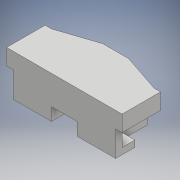
# Autodesk Inventor part: NewLaptopSupport
Saved by Autodesk Inventor 2017 (Build 210142000, 142)
## iProperties
Created: 2016-11-02
Part Number: NewLaptopSupport
Material: Generic
Document SubType Name: Modeling
Designer: Schmidty15
Density: 1 g/cm^3
Appearance: Default
Author: Schmidty15
Autodesk Inventor part; units mm, degrees
ref_plane "YZ Plane" through (0, 0, 0) normal (1, 0, 0) x (0, 1, 0)
ref_plane "XZ Plane" through (0, 0, 0) normal (0, 1, 0) x (-1, 0, 0)
ref_plane "XY Plane" through (0, 0, 0) normal (0, 0, 1) x (1, 0, 0)
sketch "Sketch1" plane through (0, 0, 0) normal (0, 1, 0) x (-1, 0, 0)
  line L0 (0, 0) -> (-160, 0)
  line L1 (-160, 0) -> (-160, 60)
  line L2 (-160, 60) -> (0, 60)
  line L3 (0, 60) -> (0, 0)
  dimension "d0" = 160
  dimension "d1" = 60
  constraints: 8 end point, 2 parallel, 1 horizontal, 1 perpendicular
  measures "d0" distance of L1.end L2.end
  measures "d1" distance of L0.end L1.end
extrude "Extrusion1" add sketch "Sketch1" along normal blind 80
sketch "Sketch2" plane through (0, 80, 0) normal (0, 1, 0) x (1, 0, 0)
  line L0 (160, 0) -> (0, 0) projected
  line L1 (160, 0) -> (150, 0)
  line L2 (150, 0) -> (150, -10)
  line L3 (150, -10) -> (160, -10)
  line L4 (160, -10) -> (160, 0)
  line L5 (160, -10) -> (0, -10)
  line L6 (0, -10) -> (0, -40)
  line L7 (0, -40) -> (160, -40)
  line L8 (160, -40) -> (160, -10)
  dimension "d4" = 10
  dimension "d5" = 10
  dimension "d6" = 160
  dimension "d7" = 30
  constraints: 16 end point, 4 parallel, 2 horizontal, 2 perpendicular
  measures "d4" distance of L3.end L2.end
  measures "d5" distance of L2.end L1.end
  measures "d6" distance of L7.end L6.end
  measures "d7" distance of L6.end L5.end
extrude "Extrusion2" cut sketch "Sketch2" against normal blind 70 contours L8 L7 L6 L5 L3
sketch "Sketch3" plane through (0, 80, 0) normal (0, 1, 0) x (1, 0, 0)
  line L0 (160, -40) -> (0, -40) projected
  line L1 (0, -40) -> (160, -40)
  line L2 (160, -40) -> (160, -50)
  line L3 (160, -50) -> (0, -50)
  line L4 (0, -50) -> (0, -40)
  point P0 (0, 0)
  dimension "d10" = 160
  dimension "d11" = 10
  constraints: 8 end point, 2 parallel, 1 horizontal, 1 perpendicular
  measures "d10" distance of L2.end L3.end
  measures "d11" distance of L1.end L2.end
extrude "Extrusion3" cut sketch "Sketch3" against normal blind 10
sketch "Sketch4" plane through (160, 10, 40) normal (0, 0, -1) x (-1, 0, 0)
  line L0 (0, 0) -> (160, 0) projected
  arc A0 (160, 0) -> (0, 0) centre (80, -23.3333) ccw
  line L1 (0, 0) -> (0, 60) projected
  line L2 (0, 0) -> (0, 60)
  line L3 (0, 60) -> (80, 60)
  line L4 (160, 60) -> (0, 60) projected
  line L5 (160, 60) -> (160, 0) projected
  line L6 (160, 0) -> (160, 60)
  line L7 (160, 60) -> (80, 60)
  point P0 (160, -10)
  constraints: 8 end point, 2 collinear, 2 point on circle, 1 centre point, 1 midpoint, 1 perpendicular, 1 tangent
extrude "Extrusion4" cut sketch "Sketch4" against normal blind 10 contours L1 L3 A0 | A0 L4 L5
sketch "Sketch5" plane through (160, 0, 0) normal (0, 0, -1) x (-1, 0, 0)
  line L0 (0, 80) -> (160, 80) projected
  line L1 (0, 80) -> (20, 80)
  line L2 (20, 80) -> (20, 30)
  line L3 (20, 30) -> (0, 30)
  line L4 (0, 30) -> (0, 80)
  line L5 (160, 10) -> (160, 80) projected
  line L6 (160, 80) -> (140, 80)
  line L7 (140, 80) -> (140, 30)
  line L8 (140, 30) -> (160, 30)
  line L9 (160, 30) -> (160, 80)
  point P0 (160, 0)
  dimension "d16" = 20
  dimension "d17" = 50
  dimension "d18" = 20
  dimension "d19" = 50
  constraints: 16 end point, 4 parallel, 2 horizontal, 2 perpendicular
  measures "d16" distance of L2.end L3.end
  measures "d17" distance of L1.end L2.end
  measures "d18" distance of L8.end L7.end
  measures "d19" distance of L7.end L6.end
extrude "Extrusion5" cut sketch "Sketch5" against normal blind 10
sketch "Sketch6" plane through (0, 80, 0) normal (0, 1, 0) x (1, 0, 0)
  line L0 (20, 0) -> (20, -10) projected
  line L1 (20, -10) -> (140, -10)
  line L2 (140, -10) -> (140, 0)
  line L3 (140, 0) -> (20, 0)
  line L4 (20, 0) -> (20, -10)
  point P0 (0, 0)
  dimension "d22" = 120
  dimension "d23" = 10
  constraints: 8 end point, 2 parallel, 1 horizontal, 1 perpendicular
  measures "d22" distance of L3.end L2.end
  measures "d23" distance of L2.end L1.end
extrude "Extrusion6" cut sketch "Sketch6" against normal blind 10
sketch "Sketch7" plane through (160, 80, 50) normal (0, 0, -1) x (-1, 0, 0)
  line L0 (0, 0) -> (0, -20)
  line L1 (0, -70) -> (0, 0) projected
  line L2 (0, -20) -> (0, 0)
  line L3 (160, 0) -> (0, 0) projected
  line L4 (0, 0) -> (60, 0)
  line L5 (60, 0) -> (0, -20)
  line L6 (0, 0) -> (160, 0) projected
  line L7 (160, 0) -> (160, -20)
  line L8 (160, 0) -> (160, -70) projected
  line L9 (160, 0) -> (100, 0)
  line L10 (100, 0) -> (160, -20)
  point P0 (160, -80)
  dimension "d26" = 20
  dimension "d27" = 60
  dimension "d28" = 20
  dimension "d29" = 60
  constraints: 14 end point, 4 point on line, 1 collinear
  measures "d26" distance of L0.start L0.end
  measures "d27" distance of L0.start L4.end
  measures "d28" distance of L3.start L7.end
  measures "d29" distance of L3.start L9.end
extrude "Extrusion7" cut sketch "Sketch7" against normal blind 10
sketch "Sketch8" plane through (140, 30, 10) normal (1, 0, 0) x (0, 0, -1)
  line L0 (10, 40) -> (0, 40) projected
  line L1 (10, 0) -> (10, 40) projected
  line L2 (0, 40) -> (10, 40)
  line L3 (10, 40) -> (10, 0)
  line L4 (10, 0) -> (0, 0)
  line L5 (0, 0) -> (0, 40)
  point P0 (10, -30)
  constraints: 8 end point, 2 parallel, 1 horizontal, 1 perpendicular
extrude "Extrusion8" cut sketch "Sketch8" against normal blind 0.5
sketch "Sketch9" plane through (20, 30, 0) normal (-1, 0, 0) x (0, 0, 1)
  line L0 (10, 40) -> (10, 0) projected
  line L1 (0, 0) -> (10, 0) projected
  line L2 (10, 40) -> (0, 40)
  line L3 (0, 40) -> (0, 0)
  line L4 (0, 0) -> (10, 0)
  line L5 (10, 0) -> (10, 40)
  point P0 (0, -30)
  constraints: 8 end point, 2 parallel, 1 horizontal, 1 perpendicular
extrude "Extrusion9" cut sketch "Sketch9" against normal blind 0.5
sketch "Sketch11" plane through (80, -13.3333, 40) normal (0, 0, -1) x (-1, 0, 0)
  line L0 (-80, 23.3333) -> (-80, 73.3333) projected
  arc A0 (80, 23.3333) -> (-80, 23.3333) centre (0, 0) ccw
  line L1 (-80, 23.3333) -> (80, 23.3333) projected
  line L2 (-80, 23.3333) -> (80, 23.3333)
  point P0 (80, 13.3333)
  constraints: 2 end point, 2 point on circle, 1 centre point, 1 horizontal
extrude "Extrusion10" cut sketch "Sketch11" against normal blind 10
sketch "Sketch12" plane through (160, 10, 50) normal (0, 0, -1) x (-1, 0, 0)
  line L0 (60, 70) -> (0, 50) projected
  line L1 (0, 0) -> (0, 50) projected
  line L2 (160, 0) -> (0, 0) projected
  line L3 (160, 50) -> (160, 0) projected
  line L4 (160, 50) -> (100, 70) projected
  line L5 (60, 70) -> (100, 70) projected
  point P0 (160, -10)
extrude "Extrusion11" cut sketch "Sketch12" against normal blind 5
sketch "Sketch13" plane through (0, 10, 0) normal (0, 1, 0) x (1, 0, 0)
  line L0 (0, -55) -> (160, -55)
  line L1 (160, -55) -> (160, -40)
  line L2 (160, -40) -> (0, -40)
  line L3 (0, -40) -> (0, -55)
  point P0 (0, 0)
  dimension "d40" = 160
  dimension "d41" = 15
  constraints: 8 end point, 2 parallel, 1 horizontal, 1 perpendicular
  measures "d40" distance of L2.end L1.end
  measures "d41" distance of L1.end L0.end
extrude "Extrusion12" add sketch "Sketch13" along normal blind 20
sketch "Sketch14" plane through (0, 30, 0) normal (0, 1, 0) x (1, 0, 0)
  line L0 (0, -40) -> (160, -40) projected
  line L1 (160, -40) -> (100, -40)
  line L2 (100, -40) -> (100, -55)
  line L3 (100, -55) -> (160, -55)
  line L4 (160, -55) -> (160, -40)
  line L5 (0, -40) -> (0, -55) projected
  line L6 (60, -55) -> (0, -55) projected
  line L7 (0, -40) -> (60, -40)
  line L8 (60, -40) -> (60, -55)
  line L9 (60, -55) -> (0, -55)
  line L10 (0, -55) -> (0, -40)
  line L11 (100, -40) -> (60, -40)
  line L12 (60, -40) -> (60, -55)
  line L13 (60, -55) -> (100, -55)
  line L14 (100, -55) -> (100, -40)
  point P0 (0, 0)
  dimension "d44" = 60
  dimension "d45" = 15
  dimension "d46" = 60
  dimension "d47" = 15
  constraints: 24 end point, 6 parallel, 3 horizontal, 3 perpendicular
  measures "d44" distance of L3.end L2.end
  measures "d45" distance of L2.end L1.end
  measures "d46" distance of L6.start L9.end
  measures "d47" distance of L7.end L6.start
extrude "Extrusion13" cut sketch "Sketch14" against normal blind 20 contours L0 L2 L13 L8
sketch "Sketch15" plane through (0, 0, 0) normal (-1, 0, 0) x (0, 0, 1)
  line L0 (40, 30) -> (55, 30) projected
  line L1 (60, 0) -> (0, 0) projected
  line L2 (40, 30) -> (60, 30)
  line L3 (60, 30) -> (60, 0)
  line L4 (60, 0) -> (40, 0)
  line L5 (40, 0) -> (40, 30)
  line L6 (55, 80) -> (55, 60) projected
  line L7 (55, 60) -> (60, 60)
  line L8 (60, 60) -> (60, 30)
  line L9 (60, 30) -> (55, 30)
  line L10 (55, 30) -> (55, 60)
  constraints: 16 end point, 4 parallel, 2 horizontal, 2 perpendicular
extrude "Extrusion14" add sketch "Sketch15" along normal blind 10
sketch "Sketch16" plane through (160, 0, 60) normal (1, 0, 0) x (0, 0, -1)
  line L0 (5, 30) -> (5, 60) projected
  line L1 (0, 0) -> (0, 60) projected
  line L2 (5, 60) -> (0, 60)
  line L3 (0, 60) -> (0, 0)
  line L4 (0, 0) -> (5, 0)
  line L5 (5, 0) -> (5, 60)
  point P0 (60, 0)
  constraints: 8 end point, 2 parallel, 1 horizontal, 1 perpendicular
extrude "Extrusion15" add sketch "Sketch16" along normal blind 10
sketch "Sketch17" plane through (-10, 0, 0) normal (-1, 0, 0) x (0, 0, 1)
  line L0 (55, 30) -> (40, 30) projected
  line L1 (55, 0) -> (55, 60) projected
  line L2 (40, 30) -> (55, 30)
  line L3 (55, 30) -> (55, 0)
  line L4 (55, 0) -> (40, 0)
  line L5 (40, 0) -> (40, 30)
  point P0 (0, 0)
  constraints: 8 end point, 2 parallel, 1 horizontal, 1 perpendicular
extrude "Extrusion16" cut sketch "Sketch17" against normal blind 10
sketch "Sketch18" plane through (60, 80, 60) normal (0, 0, 1) x (1, 0, 0)
  line L0 (100, -20) -> (40, 0) projected
  line L1 (0, 0) -> (40, 0) projected
  line L2 (0, 0) -> (-60, -20) projected
  line L3 (-60, -20) -> (-70, -20) projected
  line L4 (-70, -80) -> (-70, -20) projected
  line L5 (110, -80) -> (-70, -80) projected
  line L6 (110, -20) -> (110, -80) projected
  line L7 (100, -20) -> (110, -20) projected
  point P0 (-60, -80)
extrude "Extrusion17" add sketch "Sketch18" along normal blind 5
sketch "Sketch19" plane through (160, 0, 0) normal (0, 0, -1) x (-1, 0, 0)
  line L0 (0, 0) -> (60, 0)
  line L1 (160, 0) -> (0, 0) projected
  line L2 (60, 0) -> (100, 0)
  line L3 (100, 0) -> (100, 20)
  line L4 (100, 20) -> (60, 20)
  line L5 (60, 20) -> (60, 0)
  dimension "d58" = 60
  dimension "d59" = 40
  dimension "d60" = 20
  constraints: 10 end point, 2 parallel, 1 horizontal, 1 perpendicular, 1 point on line
  measures "d58" distance of L0.start L0.end
  measures "d59" distance of L4.end L3.end
  measures "d60" distance of L3.end L2.end
extrude "Extrusion18" cut sketch "Sketch19" against normal blind 20
sketch "Sketch20" plane through (0, 10, 0) normal (0, 1, 0) x (1, 0, 0)
  line L0 (60, 0) -> (60, -20) projected
  line L1 (100, -40) -> (100, -55) projected
  line L2 (60, -20) -> (100, -20)
  line L3 (100, -20) -> (100, -55)
  line L4 (100, -55) -> (60, -55)
  line L5 (60, -55) -> (60, -20)
  point P0 (0, 0)
  constraints: 8 end point, 2 parallel, 1 horizontal, 1 perpendicular
extrude "Extrusion19" cut sketch "Sketch20" against normal blind 5
sketch "Sketch21" plane through (0, 30, 0) normal (0, 1, 0) x (1, 0, 0)
  line L0 (0, -55) -> (0, 0) projected
  line L1 (0, -55) -> (60, -55)
  line L2 (60, -55) -> (60, -40)
  line L3 (60, -40) -> (0, -40)
  line L4 (0, -40) -> (0, -55)
  line L5 (100, -40) -> (100, -55) projected
  line L6 (160, -55) -> (100, -55) projected
  line L7 (100, -40) -> (160, -40)
  line L8 (160, -40) -> (160, -55)
  line L9 (160, -55) -> (100, -55)
  line L10 (100, -55) -> (100, -40)
  constraints: 16 end point, 4 parallel, 2 horizontal, 2 perpendicular
extrude "Extrusion20" add sketch "Sketch21" along normal blind 10
sketch "Sketch22" plane through (160, 10, 55) normal (0, 0, -1) x (-1, 0, 0)
  line L0 (0, 50) -> (60, 70) projected
  line L1 (0, -10) -> (-10, -10) projected
  line L2 (0, 50) -> (-10, 50)
  line L3 (-10, 50) -> (-10, -10)
  line L4 (-10, -10) -> (0, -10)
  line L5 (0, -10) -> (0, 50)
  line L6 (160, 50) -> (170, 50) projected
  line L7 (160, -10) -> (170, -10)
  line L8 (170, -10) -> (170, 50)
  line L9 (170, 50) -> (160, 50)
  line L10 (160, 50) -> (160, -10)
  constraints: 16 end point, 4 parallel, 2 horizontal, 2 perpendicular
extrude "Extrusion21" add sketch "Sketch22" along normal blind 15
sketch "Sketch23" plane through (0, 40, 0) normal (0, 1, 0) x (1, 0, 0)
  line L0 (160, -55) -> (160, -40) projected
  line L1 (100, -40) -> (160, -40) projected
  line L2 (160, -55) -> (100, -55)
  line L3 (100, -55) -> (100, -40)
  line L4 (100, -40) -> (160, -40)
  line L5 (160, -40) -> (160, -55)
  line L6 (0, -40) -> (60, -40) projected
  line L7 (60, -55) -> (0, -55) projected
  line L8 (60, -40) -> (0, -40)
  line L9 (0, -40) -> (0, -55)
  line L10 (0, -55) -> (60, -55)
  line L11 (60, -55) -> (60, -40)
  point P0 (0, 0)
  constraints: 16 end point, 4 parallel, 2 horizontal, 2 perpendicular
extrude "Extrusion22" cut sketch "Sketch23" against normal blind 5
body "Solid1"
